bandlabels (Autodesk Fusion 360 design; units mm, degrees)
Autodesk Fusion 360 part; units mm, degrees
(part 1 of 2)
sketch "Sketch1" plane through (0, 0, 0) normal (0, 0, 1) x (1, 0, 0)
  line L0 (-15, -10) -> (-15, 8)
  line L1 (-15, 8) -> (15, 8)
  line L2 (15, 8) -> (15, -10)
  line L3 (15, -10) -> (-15, 8) construction
  line L4 (-15, -10) -> (15, 8) construction
  line L5 (15, -10) -> (15, -16.5)
  line L6 (6.1644, -16.5) -> (-15, -16.5)
  line L7 (-15, -10) -> (-15, -16.5)
  line L8 (6, 6) -> (-6, 6)
  line L9 (-6, 6) -> (-6, -6)
  line L10 (-6, -6) -> (6, -6)
  line L11 (6, -6) -> (6, 6)
  line L12 (6, 6) -> (-6, -6) construction
  line L13 (-6, 6) -> (6, -6) construction
  circle A0 centre (-11.792, 0) radius 1.75
  circle A1 centre (11.792, 0) radius 1.75
  line L14 (-15, -16.5) -> (15, -16.5)
  circle A2 centre (-11.792, -26) radius 1.75
  line L15 (-6, -32) -> (6, -32)
  line L16 (-6, -20) -> (-6, -32)
  line L17 (15, -36) -> (15, -42.5)
  line L18 (15, -18) -> (15, -36)
  line L19 (6, -32) -> (6, -20)
  line L20 (15, -36) -> (-15, -18) construction
  line L21 (-6, -20) -> (6, -32) construction
  line L22 (-15, -36) -> (15, -18) construction
  line L23 (-15, -36) -> (-15, -18)
  line L24 (6, -20) -> (-6, -20)
  line L25 (-15, -42.5) -> (15, -42.5)
  line L26 (6, -20) -> (-6, -32) construction
  circle A3 centre (11.792, -26) radius 1.75
  line L27 (-15, -36) -> (-15, -42.5)
  line L28 (6.1644, -42.5) -> (-15, -42.5)
  line L29 (-15, -18) -> (15, -18)
  line L30 (-48, -16.5) -> (-18, -16.5)
  line L31 (-18, -10) -> (-18, -16.5)
  circle A4 centre (-21.208, 0) radius 1.75
  line L32 (-27, -6) -> (-27, 6)
  line L33 (-27, 6) -> (-39, -6) construction
  line L34 (-48, -10) -> (-18, 8) construction
  line L35 (-39, 6) -> (-27, -6) construction
  circle A5 centre (-44.792, 0) radius 1.75
  line L36 (-18, -10) -> (-48, 8) construction
  line L37 (-48, -10) -> (-48, -16.5)
  line L38 (-39, 6) -> (-39, -6)
  line L39 (-27, 6) -> (-39, 6)
  line L40 (-26.8356, -16.5) -> (-48, -16.5)
  line L41 (-18, 8) -> (-18, -10)
  line L42 (-39, -6) -> (-27, -6)
  line L43 (-48, 8) -> (-18, 8)
  line L44 (-48, -10) -> (-48, 8)
  line L45 (-18, -36) -> (-48, -18) construction
  line L46 (-48, -36) -> (-48, -18)
  line L47 (-48, -42.5) -> (-18, -42.5)
  line L48 (-27, -32) -> (-27, -20)
  line L49 (-48, -36) -> (-48, -42.5)
  line L50 (-27, -20) -> (-39, -32) construction
  circle A6 centre (-44.792, -26) radius 1.75
  line L51 (-48, -18) -> (-18, -18)
  line L52 (-39, -20) -> (-39, -32)
  line L53 (-39, -20) -> (-27, -32) construction
  line L54 (-39, -32) -> (-27, -32)
  line L55 (-27, -20) -> (-39, -20)
  circle A7 centre (-21.208, -26) radius 1.75
  line L56 (-18, -18) -> (-18, -36)
  line L57 (-26.8356, -42.5) -> (-48, -42.5)
  line L58 (-18, -36) -> (-18, -42.5)
  line L59 (-48, -36) -> (-18, -18) construction
  line L60 (38, -6) -> (38, 6)
  line L61 (26, 6) -> (38, -6) construction
  line L62 (38, 6) -> (26, -6) construction
  circle A8 centre (20.208, 0) radius 1.75
  circle A9 centre (43.792, 0) radius 1.75
  line L63 (38, 6) -> (26, 6)
  line L64 (26, -6) -> (38, -6)
  line L65 (47, -10) -> (47, -16.5)
  line L66 (17, 8) -> (47, 8)
  line L67 (17, -10) -> (47, 8) construction
  line L68 (47, 8) -> (47, -10)
  line L69 (47, -10) -> (17, 8) construction
  line L70 (17, -16.5) -> (47, -16.5)
  line L71 (17, -10) -> (17, -16.5)
  line L72 (17, -10) -> (17, 8)
  line L73 (38.1644, -16.5) -> (17, -16.5)
  line L74 (26, 6) -> (26, -6)
  line L75 (17, -36) -> (47, -18) construction
  line L76 (47, -36) -> (17, -18) construction
  line L77 (47, -36) -> (47, -42.5)
  line L78 (38.1644, -42.5) -> (17, -42.5)
  line L79 (17, -36) -> (17, -42.5)
  circle A10 centre (43.792, -26) radius 1.75
  line L80 (17, -18) -> (47, -18)
  line L81 (38, -32) -> (38, -20)
  circle A11 centre (20.208, -26) radius 1.75
  line L82 (38, -20) -> (26, -32) construction
  line L83 (26, -32) -> (38, -32)
  line L84 (26, -20) -> (26, -32)
  line L85 (26, -20) -> (38, -32) construction
  line L86 (38, -20) -> (26, -20)
  line L87 (47, -18) -> (47, -36)
  line L88 (17, -36) -> (17, -18)
  line L89 (17, -42.5) -> (47, -42.5)
  line L90 (-18, -63) -> (-18, -69.5)
  line L91 (-27, -47) -> (-39, -59) construction
  line L92 (-48, -63) -> (-18, -45) construction
  circle A12 centre (-21.208, -53) radius 1.75
  line L93 (-48, -63) -> (-48, -45)
  line L94 (-48, -69.5) -> (-18, -69.5)
  line L95 (-18, -63) -> (-48, -45) construction
  line L96 (-39, -47) -> (-39, -59)
  line L97 (-26.8356, -69.5) -> (-48, -69.5)
  line L98 (-48, -45) -> (-18, -45)
  line L99 (-27, -47) -> (-39, -47)
  line L100 (-18, -45) -> (-18, -63)
  circle A13 centre (-44.792, -53) radius 1.75
  line L101 (-48, -63) -> (-48, -69.5)
  line L102 (-27, -59) -> (-27, -47)
  line L103 (-39, -47) -> (-27, -59) construction
  line L104 (-39, -59) -> (-27, -59)
  line L105 (-42.7356, -14.4017) -> (-42.7356, -14.9918)
  line L106 (-42.7356, -14.9918) -> (-46.0406, -14.9918)
  spline S0 degree 2 poles (-46.0406, -14.9918) (-46.0474, -14.7701) (-45.9689, -14.5655) knots 0 0 0 1 1 1
  spline S1 degree 2 poles (-45.9689, -14.5655) (-45.8427, -14.2278) (-45.5648, -13.9004) knots 0 0 0 1 1 1
  spline S2 degree 2 poles (-45.5648, -13.9004) (-45.2868, -13.573) (-44.7616, -13.1432) knots 0 0 0 1 1 1
  spline S3 degree 2 poles (-44.7616, -13.1432) (-43.9464, -12.4747) (-43.6599, -12.0842) knots 0 0 0 1 1 1
  spline S4 degree 2 poles (-43.6599, -12.0842) (-43.3734, -11.6937) (-43.3734, -11.3458) knots 0 0 0 1 1 1
  spline S5 degree 2 poles (-43.3734, -11.3458) (-43.3734, -10.9809) (-43.6344, -10.7302) knots 0 0 0 1 1 1
  spline S6 degree 2 poles (-43.6344, -10.7302) (-43.8953, -10.4795) (-44.3148, -10.4795) knots 0 0 0 1 1 1
  spline S7 degree 2 poles (-44.3148, -10.4795) (-44.7582, -10.4795) (-45.0242, -10.7455) knots 0 0 0 1 1 1
  spline S8 degree 2 poles (-45.0242, -10.7455) (-45.2902, -11.0116) (-45.2936, -11.4822) knots 0 0 0 1 1 1
  line L107 (-45.2936, -11.4822) -> (-45.9246, -11.4174)
  spline S9 degree 2 poles (-45.9246, -11.4174) (-45.8598, -10.7114) (-45.4369, -10.3414) knots 0 0 0 1 1 1
  spline S10 degree 2 poles (-45.4369, -10.3414) (-45.014, -9.9713) (-44.3011, -9.9713) knots 0 0 0 1 1 1
  spline S11 degree 2 poles (-44.3011, -9.9713) (-43.5815, -9.9713) (-43.162, -10.3704) knots 0 0 0 1 1 1
  spline S12 degree 2 poles (-43.162, -10.3704) (-42.7425, -10.7694) (-42.7425, -11.3594) knots 0 0 0 1 1 1
  spline S13 degree 2 poles (-42.7425, -11.3594) (-42.7425, -11.6596) (-42.8653, -11.9495) knots 0 0 0 1 1 1
  spline S14 degree 2 poles (-42.8653, -11.9495) (-42.988, -12.2394) (-43.2728, -12.56) knots 0 0 0 1 1 1
  spline S15 degree 2 poles (-43.2728, -12.56) (-43.5576, -12.8806) (-44.2193, -13.4399) knots 0 0 0 1 1 1
  spline S16 degree 2 poles (-44.2193, -13.4399) (-44.7718, -13.9038) (-44.9287, -14.0692) knots 0 0 0 1 1 1
  spline S17 degree 2 poles (-44.9287, -14.0692) (-45.0856, -14.2346) (-45.1879, -14.4017) knots 0 0 0 1 1 1
  line L108 (-45.1879, -14.4017) -> (-42.7356, -14.4017)
  spline S18 degree 2 poles (-42.0774, -12.5259) (-42.0774, -11.6391) (-41.8949, -11.0985) knots 0 0 0 1 1 1
  spline S19 degree 2 poles (-41.8949, -11.0985) (-41.7125, -10.5579) (-41.3526, -10.2646) knots 0 0 0 1 1 1
  spline S20 degree 2 poles (-41.3526, -10.2646) (-40.9928, -9.9713) (-40.4471, -9.9713) knots 0 0 0 1 1 1
  spline S21 degree 2 poles (-40.4471, -9.9713) (-40.0447, -9.9713) (-39.7411, -10.1333) knots 0 0 0 1 1 1
  spline S22 degree 2 poles (-39.7411, -10.1333) (-39.4376, -10.2953) (-39.2397, -10.6006) knots 0 0 0 1 1 1
  spline S23 degree 2 poles (-39.2397, -10.6006) (-39.0419, -10.9058) (-38.9294, -11.3441) knots 0 0 0 1 1 1
  spline S24 degree 2 poles (-38.9294, -11.3441) (-38.8168, -11.7824) (-38.8168, -12.5259) knots 0 0 0 1 1 1
  spline S25 degree 2 poles (-38.8168, -12.5259) (-38.8168, -13.4058) (-38.9976, -13.9464) knots 0 0 0 1 1 1
  spline S26 degree 2 poles (-38.9976, -13.9464) (-39.1784, -14.487) (-39.5382, -14.782) knots 0 0 0 1 1 1
  spline S27 degree 2 poles (-39.5382, -14.782) (-39.898, -15.077) (-40.4471, -15.077) knots 0 0 0 1 1 1
  spline S28 degree 2 poles (-40.4471, -15.077) (-41.1702, -15.077) (-41.5829, -14.5586) knots 0 0 0 1 1 1
  spline S29 degree 2 poles (-41.5829, -14.5586) (-42.0774, -13.9345) (-42.0774, -12.5259) knots 0 0 0 1 1 1
  spline S30 degree 2 poles (-41.4464, -12.5259) (-41.4464, -13.7571) (-41.1582, -14.1647) knots 0 0 0 1 1 1
  spline S31 degree 2 poles (-41.1582, -14.1647) (-40.87, -14.5723) (-40.4471, -14.5723) knots 0 0 0 1 1 1
  spline S32 degree 2 poles (-40.4471, -14.5723) (-40.0242, -14.5723) (-39.736, -14.163) knots 0 0 0 1 1 1
  spline S33 degree 2 poles (-39.736, -14.163) (-39.4478, -13.7537) (-39.4478, -12.5259) knots 0 0 0 1 1 1
  spline S34 degree 2 poles (-39.4478, -12.5259) (-39.4478, -11.2912) (-39.736, -10.8854) knots 0 0 0 1 1 1
  spline S35 degree 2 poles (-39.736, -10.8854) (-40.0242, -10.4795) (-40.4539, -10.4795) knots 0 0 0 1 1 1
  spline S36 degree 2 poles (-40.4539, -10.4795) (-40.8769, -10.4795) (-41.1292, -10.8376) knots 0 0 0 1 1 1
  spline S37 degree 2 poles (-41.1292, -10.8376) (-41.4464, -11.2946) (-41.4464, -12.5259) knots 0 0 0 1 1 1
  line L109 (-38.4826, -15.077) -> (-37.0331, -9.9065)
  line L110 (-37.0331, -9.9065) -> (-36.5419, -9.9065)
  line L111 (-36.5419, -9.9065) -> (-37.988, -15.077)
  line L112 (-37.988, -15.077) -> (-38.4826, -15.077)
  line L113 (-34.2841, -14.9918) -> (-34.2841, -13.7946)
  line L114 (-34.2841, -13.7946) -> (-36.4532, -13.7946)
  line L115 (-36.4532, -13.7946) -> (-36.4532, -13.2319)
  line L116 (-36.4532, -13.2319) -> (-34.1715, -9.9918)
  line L117 (-34.1715, -9.9918) -> (-33.6702, -9.9918)
  line L118 (-33.6702, -9.9918) -> (-33.6702, -13.2319)
  line L119 (-33.6702, -13.2319) -> (-32.9949, -13.2319)
  line L120 (-32.9949, -13.2319) -> (-32.9949, -13.7946)
  line L121 (-32.9949, -13.7946) -> (-33.6702, -13.7946)
  line L122 (-33.6702, -13.7946) -> (-33.6702, -14.9918)
  line L123 (-33.6702, -14.9918) -> (-34.2841, -14.9918)
  line L124 (-34.2841, -13.2319) -> (-34.2841, -10.9775)
  line L125 (-34.2841, -10.9775) -> (-35.8496, -13.2319)
  line L126 (-35.8496, -13.2319) -> (-34.2841, -13.2319)
  spline S38 degree 2 poles (-32.3673, -12.5259) (-32.3673, -11.6391) (-32.1848, -11.0985) knots 0 0 0 1 1 1
  spline S39 degree 2 poles (-32.1848, -11.0985) (-32.0024, -10.5579) (-31.6425, -10.2646) knots 0 0 0 1 1 1
  spline S40 degree 2 poles (-31.6425, -10.2646) (-31.2827, -9.9713) (-30.737, -9.9713) knots 0 0 0 1 1 1
  spline S41 degree 2 poles (-30.737, -9.9713) (-30.3346, -9.9713) (-30.031, -10.1333) knots 0 0 0 1 1 1
  spline S42 degree 2 poles (-30.031, -10.1333) (-29.7275, -10.2953) (-29.5296, -10.6006) knots 0 0 0 1 1 1
  spline S43 degree 2 poles (-29.5296, -10.6006) (-29.3318, -10.9058) (-29.2193, -11.3441) knots 0 0 0 1 1 1
  spline S44 degree 2 poles (-29.2193, -11.3441) (-29.1067, -11.7824) (-29.1067, -12.5259) knots 0 0 0 1 1 1
  spline S45 degree 2 poles (-29.1067, -12.5259) (-29.1067, -13.4058) (-29.2875, -13.9464) knots 0 0 0 1 1 1
  spline S46 degree 2 poles (-29.2875, -13.9464) (-29.4683, -14.487) (-29.8281, -14.782) knots 0 0 0 1 1 1
  spline S47 degree 2 poles (-29.8281, -14.782) (-30.1879, -15.077) (-30.737, -15.077) knots 0 0 0 1 1 1
  spline S48 degree 2 poles (-30.737, -15.077) (-31.4601, -15.077) (-31.8728, -14.5586) knots 0 0 0 1 1 1
  spline S49 degree 2 poles (-31.8728, -14.5586) (-32.3673, -13.9345) (-32.3673, -12.5259) knots 0 0 0 1 1 1
  spline S50 degree 2 poles (-31.7363, -12.5259) (-31.7363, -13.7571) (-31.4481, -14.1647) knots 0 0 0 1 1 1
  spline S51 degree 2 poles (-31.4481, -14.1647) (-31.1599, -14.5723) (-30.737, -14.5723) knots 0 0 0 1 1 1
  spline S52 degree 2 poles (-30.737, -14.5723) (-30.3141, -14.5723) (-30.0259, -14.163) knots 0 0 0 1 1 1
  spline S53 degree 2 poles (-30.0259, -14.163) (-29.7377, -13.7537) (-29.7377, -12.5259) knots 0 0 0 1 1 1
  spline S54 degree 2 poles (-29.7377, -12.5259) (-29.7377, -11.2912) (-30.0259, -10.8854) knots 0 0 0 1 1 1
  spline S55 degree 2 poles (-30.0259, -10.8854) (-30.3141, -10.4795) (-30.7438, -10.4795) knots 0 0 0 1 1 1
  spline S56 degree 2 poles (-30.7438, -10.4795) (-31.1668, -10.4795) (-31.4191, -10.8376) knots 0 0 0 1 1 1
  spline S57 degree 2 poles (-31.4191, -10.8376) (-31.7363, -11.2946) (-31.7363, -12.5259) knots 0 0 0 1 1 1
  line L127 (-28.7725, -15.077) -> (-27.323, -9.9065)
  line L128 (-27.323, -9.9065) -> (-26.8318, -9.9065)
  line L129 (-26.8318, -9.9065) -> (-28.2779, -15.077)
  line L130 (-28.2779, -15.077) -> (-28.7725, -15.077)
  line L131 (-23.3564, -11.2162) -> (-23.9669, -11.264)
  spline S58 degree 2 poles (-23.9669, -11.264) (-24.0487, -10.9024) (-24.1988, -10.7387) knots 0 0 0 1 1 1
  spline S59 degree 2 poles (-24.1988, -10.7387) (-24.4478, -10.4761) (-24.8127, -10.4761) knots 0 0 0 1 1 1
  spline S60 degree 2 poles (-24.8127, -10.4761) (-25.106, -10.4761) (-25.3277, -10.6398) knots 0 0 0 1 1 1
  spline S61 degree 2 poles (-25.3277, -10.6398) (-25.6176, -10.8513) (-25.7848, -11.2571) knots 0 0 0 1 1 1
  spline S62 degree 2 poles (-25.7848, -11.2571) (-25.9519, -11.663) (-25.9587, -12.4133) knots 0 0 0 1 1 1
  spline S63 degree 2 poles (-25.9587, -12.4133) (-25.737, -12.0757) (-25.4164, -11.912) knots 0 0 0 1 1 1
  spline S64 degree 2 poles (-25.4164, -11.912) (-25.0958, -11.7483) (-24.7445, -11.7483) knots 0 0 0 1 1 1
  spline S65 degree 2 poles (-24.7445, -11.7483) (-24.1306, -11.7483) (-23.6992, -12.2002) knots 0 0 0 1 1 1
  spline S66 degree 2 poles (-23.6992, -12.2002) (-23.2677, -12.6521) (-23.2677, -13.3683) knots 0 0 0 1 1 1
  spline S67 degree 2 poles (-23.2677, -13.3683) (-23.2677, -13.839) (-23.4706, -14.2431) knots 0 0 0 1 1 1
  spline S68 degree 2 poles (-23.4706, -14.2431) (-23.6736, -14.6473) (-24.0283, -14.8622) knots 0 0 0 1 1 1
  spline S69 degree 2 poles (-24.0283, -14.8622) (-24.383, -15.077) (-24.8332, -15.077) knots 0 0 0 1 1 1
  spline S70 degree 2 poles (-24.8332, -15.077) (-25.6006, -15.077) (-26.0849, -14.5126) knots 0 0 0 1 1 1
  spline S71 degree 2 poles (-26.0849, -14.5126) (-26.5692, -13.9481) (-26.5692, -12.6521) knots 0 0 0 1 1 1
  spline S72 degree 2 poles (-26.5692, -12.6521) (-26.5692, -11.2026) (-26.0337, -10.5443) knots 0 0 0 1 1 1
  spline S73 degree 2 poles (-26.0337, -10.5443) (-25.5665, -9.9713) (-24.7752, -9.9713) knots 0 0 0 1 1 1
  spline S74 degree 2 poles (-24.7752, -9.9713) (-24.1852, -9.9713) (-23.8083, -10.3022) knots 0 0 0 1 1 1
  spline S75 degree 2 poles (-23.8083, -10.3022) (-23.4314, -10.633) (-23.3564, -11.2162) knots 0 0 0 1 1 1
  spline S76 degree 2 poles (-25.8632, -13.3717) (-25.8632, -13.6889) (-25.7285, -13.9788) knots 0 0 0 1 1 1
  spline S77 degree 2 poles (-25.7285, -13.9788) (-25.5938, -14.2687) (-25.3516, -14.4205) knots 0 0 0 1 1 1
  spline S78 degree 2 poles (-25.3516, -14.4205) (-25.1095, -14.5723) (-24.8434, -14.5723) knots 0 0 0 1 1 1
  spline S79 degree 2 poles (-24.8434, -14.5723) (-24.4546, -14.5723) (-24.1749, -14.2585) knots 0 0 0 1 1 1
  spline S80 degree 2 poles (-24.1749, -14.2585) (-23.8953, -13.9447) (-23.8953, -13.4058) knots 0 0 0 1 1 1
  spline S81 degree 2 poles (-23.8953, -13.4058) (-23.8953, -12.8874) (-24.1715, -12.589) knots 0 0 0 1 1 1
  spline S82 degree 2 poles (-24.1715, -12.589) (-24.4478, -12.2906) (-24.8673, -12.2906) knots 0 0 0 1 1 1
  spline S83 degree 2 poles (-24.8673, -12.2906) (-25.2834, -12.2906) (-25.5733, -12.589) knots 0 0 0 1 1 1
  spline S84 degree 2 poles (-25.5733, -12.589) (-25.8632, -12.8874) (-25.8632, -13.3717) knots 0 0 0 1 1 1
  spline S85 degree 2 poles (-22.6572, -12.5259) (-22.6572, -11.6391) (-22.4747, -11.0985) knots 0 0 0 1 1 1
  spline S86 degree 2 poles (-22.4747, -11.0985) (-22.2923, -10.5579) (-21.9324, -10.2646) knots 0 0 0 1 1 1
  spline S87 degree 2 poles (-21.9324, -10.2646) (-21.5726, -9.9713) (-21.0269, -9.9713) knots 0 0 0 1 1 1
  spline S88 degree 2 poles (-21.0269, -9.9713) (-20.6245, -9.9713) (-20.3209, -10.1333) knots 0 0 0 1 1 1
  spline S89 degree 2 poles (-20.3209, -10.1333) (-20.0174, -10.2953) (-19.8196, -10.6006) knots 0 0 0 1 1 1
  spline S90 degree 2 poles (-19.8196, -10.6006) (-19.6217, -10.9058) (-19.5092, -11.3441) knots 0 0 0 1 1 1
  spline S91 degree 2 poles (-19.5092, -11.3441) (-19.3966, -11.7824) (-19.3966, -12.5259) knots 0 0 0 1 1 1
  spline S92 degree 2 poles (-19.3966, -12.5259) (-19.3966, -13.4058) (-19.5774, -13.9464) knots 0 0 0 1 1 1
  spline S93 degree 2 poles (-19.5774, -13.9464) (-19.7582, -14.487) (-20.118, -14.782) knots 0 0 0 1 1 1
  spline S94 degree 2 poles (-20.118, -14.782) (-20.4778, -15.077) (-21.0269, -15.077) knots 0 0 0 1 1 1
  spline S95 degree 2 poles (-21.0269, -15.077) (-21.75, -15.077) (-22.1627, -14.5586) knots 0 0 0 1 1 1
  spline S96 degree 2 poles (-22.1627, -14.5586) (-22.6572, -13.9345) (-22.6572, -12.5259) knots 0 0 0 1 1 1
  spline S97 degree 2 poles (-22.0262, -12.5259) (-22.0262, -13.7571) (-21.738, -14.1647) knots 0 0 0 1 1 1
  spline S98 degree 2 poles (-21.738, -14.1647) (-21.4498, -14.5723) (-21.0269, -14.5723) knots 0 0 0 1 1 1
  spline S99 degree 2 poles (-21.0269, -14.5723) (-20.604, -14.5723) (-20.3158, -14.163) knots 0 0 0 1 1 1
  spline S100 degree 2 poles (-20.3158, -14.163) (-20.0276, -13.7537) (-20.0276, -12.5259) knots 0 0 0 1 1 1
  spline S101 degree 2 poles (-20.0276, -12.5259) (-20.0276, -11.2912) (-20.3158, -10.8854) knots 0 0 0 1 1 1
  spline S102 degree 2 poles (-20.3158, -10.8854) (-20.604, -10.4795) (-21.0337, -10.4795) knots 0 0 0 1 1 1
  spline S103 degree 2 poles (-21.0337, -10.4795) (-21.4567, -10.4795) (-21.709, -10.8376) knots 0 0 0 1 1 1
  spline S104 degree 2 poles (-21.709, -10.8376) (-22.0262, -11.2946) (-22.0262, -12.5259) knots 0 0 0 1 1 1
  line L132 (-5.9416, -14.912) -> (-6.5555, -14.912)
  line L133 (-6.5555, -14.912) -> (-6.5555, -11)
  spline S105 degree 2 poles (-6.5555, -11) (-6.7772, -11.2115) (-7.137, -11.4229) knots 0 0 0 1 1 1
  spline S106 degree 2 poles (-7.137, -11.4229) (-7.4968, -11.6344) (-7.7833, -11.7401) knots 0 0 0 1 1 1
  line L134 (-7.7833, -11.7401) -> (-7.7833, -11.1467)
  spline S107 degree 2 poles (-7.7833, -11.1467) (-7.2683, -10.9045) (-6.8829, -10.56) knots 0 0 0 1 1 1
  spline S108 degree 2 poles (-6.8829, -10.56) (-6.4975, -10.2156) (-6.3372, -9.8916) knots 0 0 0 1 1 1
  line L135 (-6.3372, -9.8916) -> (-5.9416, -9.8916)
  line L136 (-5.9416, -9.8916) -> (-5.9416, -14.912)
  line L137 (-4.3693, -13.6023) -> (-3.7246, -13.5478)
  spline S109 degree 2 poles (-3.7246, -13.5478) (-3.653, -14.0184) (-3.3921, -14.2555) knots 0 0 0 1 1 1
  spline S110 degree 2 poles (-3.3921, -14.2555) (-3.1312, -14.4925) (-2.7628, -14.4925) knots 0 0 0 1 1 1
  spline S111 degree 2 poles (-2.7628, -14.4925) (-2.3195, -14.4925) (-2.0125, -14.1583) knots 0 0 0 1 1 1
  spline S112 degree 2 poles (-2.0125, -14.1583) (-1.7055, -13.824) (-1.7055, -13.2715) knots 0 0 0 1 1 1
  spline S113 degree 2 poles (-1.7055, -13.2715) (-1.7055, -12.7463) (-2.0006, -12.4427) knots 0 0 0 1 1 1
  spline S114 degree 2 poles (-2.0006, -12.4427) (-2.2956, -12.1392) (-2.7731, -12.1392) knots 0 0 0 1 1 1
  spline S115 degree 2 poles (-2.7731, -12.1392) (-3.0698, -12.1392) (-3.3085, -12.2739) knots 0 0 0 1 1 1
  spline S116 degree 2 poles (-3.3085, -12.2739) (-3.5473, -12.4086) (-3.6837, -12.6235) knots 0 0 0 1 1 1
  line L138 (-3.6837, -12.6235) -> (-4.2601, -12.5484)
  line L139 (-4.2601, -12.5484) -> (-3.7758, -9.9802)
  line L140 (-3.7758, -9.9802) -> (-1.2894, -9.9802)
  line L141 (-1.2894, -9.9802) -> (-1.2894, -10.5669)
  line L142 (-1.2894, -10.5669) -> (-3.2847, -10.5669)
  line L143 (-3.2847, -10.5669) -> (-3.5541, -11.9107)
  spline S117 degree 2 poles (-3.5541, -11.9107) (-3.1039, -11.5969) (-2.6094, -11.5969) knots 0 0 0 1 1 1
  spline S118 degree 2 poles (-2.6094, -11.5969) (-1.9545, -11.5969) (-1.5043, -12.0505) knots 0 0 0 1 1 1
  spline S119 degree 2 poles (-1.5043, -12.0505) (-1.0541, -12.5041) (-1.0541, -13.2169) knots 0 0 0 1 1 1
  spline S120 degree 2 poles (-1.0541, -13.2169) (-1.0541, -13.8957) (-1.4497, -14.3902) knots 0 0 0 1 1 1
  spline S121 degree 2 poles (-1.4497, -14.3902) (-1.9307, -14.9973) (-2.7628, -14.9973) knots 0 0 0 1 1 1
  spline S122 degree 2 poles (-2.7628, -14.9973) (-3.445, -14.9973) (-3.8764, -14.6153) knots 0 0 0 1 1 1
  spline S123 degree 2 poles (-3.8764, -14.6153) (-4.3079, -14.2333) (-4.3693, -13.6023) knots 0 0 0 1 1 1
  line L144 (1.6266, -14.912) -> (1.6266, -11.2899)
  line L145 (1.6266, -11.2899) -> (2.1758, -11.2899)
  line L146 (2.1758, -11.2899) -> (2.1758, -11.7981)
  spline S124 degree 2 poles (2.1758, -11.7981) (2.3463, -11.5321) (2.6294, -11.3701) knots 0 0 0 1 1 1
  spline S125 degree 2 poles (2.6294, -11.3701) (2.9125, -11.2081) (3.274, -11.2081) knots 0 0 0 1 1 1
  spline S126 degree 2 poles (3.274, -11.2081) (3.6764, -11.2081) (3.9339, -11.3752) knots 0 0 0 1 1 1
  spline S127 degree 2 poles (3.9339, -11.3752) (4.1915, -11.5423) (4.2972, -11.8424) knots 0 0 0 1 1 1
  spline S128 degree 2 poles (4.2972, -11.8424) (4.7269, -11.2081) (5.4159, -11.2081) knots 0 0 0 1 1 1
  spline S129 degree 2 poles (5.4159, -11.2081) (5.9548, -11.2081) (6.2447, -11.5065) knots 0 0 0 1 1 1
  spline S130 degree 2 poles (6.2447, -11.5065) (6.5346, -11.8049) (6.5346, -12.4257) knots 0 0 0 1 1 1
  line L147 (6.5346, -12.4257) -> (6.5346, -14.912)
  line L148 (6.5346, -14.912) -> (5.9241, -14.912)
  line L149 (5.9241, -14.912) -> (5.9241, -12.6303)
  spline S131 degree 2 poles (5.9241, -12.6303) (5.9241, -12.262) (5.8644, -12.1) knots 0 0 0 1 1 1
  spline S132 degree 2 poles (5.8644, -12.1) (5.8047, -11.9379) (5.6478, -11.839) knots 0 0 0 1 1 1
  spline S133 degree 2 poles (5.6478, -11.839) (5.4909, -11.7401) (5.2794, -11.7401) knots 0 0 0 1 1 1
  spline S134 degree 2 poles (5.2794, -11.7401) (4.8975, -11.7401) (4.6451, -11.9942) knots 0 0 0 1 1 1
  spline S135 degree 2 poles (4.6451, -11.9942) (4.3927, -12.2483) (4.3927, -12.8077) knots 0 0 0 1 1 1
  line L150 (4.3927, -12.8077) -> (4.3927, -14.912)
  line L151 (4.3927, -14.912) -> (3.7788, -14.912)
  line L152 (3.7788, -14.912) -> (3.7788, -12.5587)
  spline S136 degree 2 poles (3.7788, -12.5587) (3.7788, -12.1494) (3.6287, -11.9448) knots 0 0 0 1 1 1
  spline S137 degree 2 poles (3.6287, -11.9448) (3.4786, -11.7401) (3.1376, -11.7401) knots 0 0 0 1 1 1
  spline S138 degree 2 poles (3.1376, -11.7401) (2.8784, -11.7401) (2.6584, -11.8766) knots 0 0 0 1 1 1
  spline S139 degree 2 poles (2.6584, -11.8766) (2.4384, -12.013) (2.3395, -12.2756) knots 0 0 0 1 1 1
  spline S140 degree 2 poles (2.3395, -12.2756) (2.2406, -12.5382) (2.2406, -13.0328) knots 0 0 0 1 1 1
  line L153 (2.2406, -13.0328) -> (2.2406, -14.912)
  line L154 (2.2406, -14.912) -> (1.6266, -14.912)
  line L155 (26.0584, -14.912) -> (25.4445, -14.912)
  line L156 (25.4445, -14.912) -> (25.4445, -11)
  spline S141 degree 2 poles (25.4445, -11) (25.2228, -11.2115) (24.863, -11.4229) knots 0 0 0 1 1 1
  spline S142 degree 2 poles (24.863, -11.4229) (24.5032, -11.6344) (24.2167, -11.7401) knots 0 0 0 1 1 1
  line L157 (24.2167, -11.7401) -> (24.2167, -11.1467)
  spline S143 degree 2 poles (24.2167, -11.1467) (24.7317, -10.9045) (25.1171, -10.56) knots 0 0 0 1 1 1
  spline S144 degree 2 poles (25.1171, -10.56) (25.5025, -10.2156) (25.6628, -9.8916) knots 0 0 0 1 1 1
  line L158 (25.6628, -9.8916) -> (26.0584, -9.8916)
  line L159 (26.0584, -9.8916) -> (26.0584, -14.912)
  line L160 (30.8572, -14.322) -> (30.8572, -14.912)
  line L161 (30.8572, -14.912) -> (27.5523, -14.912)
  spline S145 degree 2 poles (27.5523, -14.912) (27.5455, -14.6903) (27.6239, -14.4857) knots 0 0 0 1 1 1
  spline S146 degree 2 poles (27.6239, -14.4857) (27.7501, -14.148) (28.0281, -13.8206) knots 0 0 0 1 1 1
  spline S147 degree 2 poles (28.0281, -13.8206) (28.306, -13.4932) (28.8313, -13.0635) knots 0 0 0 1 1 1
  spline S148 degree 2 poles (28.8313, -13.0635) (29.6464, -12.395) (29.9329, -12.0045) knots 0 0 0 1 1 1
  spline S149 degree 2 poles (29.9329, -12.0045) (30.2194, -11.6139) (30.2194, -11.266) knots 0 0 0 1 1 1
  spline S150 degree 2 poles (30.2194, -11.266) (30.2194, -10.9011) (29.9585, -10.6504) knots 0 0 0 1 1 1
  spline S151 degree 2 poles (29.9585, -10.6504) (29.6976, -10.3997) (29.2781, -10.3997) knots 0 0 0 1 1 1
  spline S152 degree 2 poles (29.2781, -10.3997) (28.8347, -10.3997) (28.5687, -10.6658) knots 0 0 0 1 1 1
  spline S153 degree 2 poles (28.5687, -10.6658) (28.3026, -10.9318) (28.2992, -11.4025) knots 0 0 0 1 1 1
  line L162 (28.2992, -11.4025) -> (27.6683, -11.3377)
  spline S154 degree 2 poles (27.6683, -11.3377) (27.7331, -10.6317) (28.156, -10.2616) knots 0 0 0 1 1 1
  spline S155 degree 2 poles (28.156, -10.2616) (28.5789, -9.8916) (29.2917, -9.8916) knots 0 0 0 1 1 1
  spline S156 degree 2 poles (29.2917, -9.8916) (30.0114, -9.8916) (30.4309, -10.2906) knots 0 0 0 1 1 1
  spline S157 degree 2 poles (30.4309, -10.2906) (30.8504, -10.6896) (30.8504, -11.2797) knots 0 0 0 1 1 1
  spline S158 degree 2 poles (30.8504, -11.2797) (30.8504, -11.5798) (30.7276, -11.8697) knots 0 0 0 1 1 1
  spline S159 degree 2 poles (30.7276, -11.8697) (30.6048, -12.1596) (30.32, -12.4802) knots 0 0 0 1 1 1
  spline S160 degree 2 poles (30.32, -12.4802) (30.0352, -12.8008) (29.3736, -13.3602) knots 0 0 0 1 1 1
  spline S161 degree 2 poles (29.3736, -13.3602) (28.8211, -13.824) (28.6642, -13.9894) knots 0 0 0 1 1 1
  spline S162 degree 2 poles (28.6642, -13.9894) (28.5073, -14.1549) (28.405, -14.322) knots 0 0 0 1 1 1
  line L163 (28.405, -14.322) -> (30.8572, -14.322)
  line L164 (33.6266, -14.912) -> (33.6266, -11.2899)
  line L165 (33.6266, -11.2899) -> (34.1758, -11.2899)
  line L166 (34.1758, -11.2899) -> (34.1758, -11.7981)
  spline S163 degree 2 poles (34.1758, -11.7981) (34.3463, -11.5321) (34.6294, -11.3701) knots 0 0 0 1 1 1
  spline S164 degree 2 poles (34.6294, -11.3701) (34.9125, -11.2081) (35.274, -11.2081) knots 0 0 0 1 1 1
  spline S165 degree 2 poles (35.274, -11.2081) (35.6764, -11.2081) (35.9339, -11.3752) knots 0 0 0 1 1 1
  spline S166 degree 2 poles (35.9339, -11.3752) (36.1915, -11.5423) (36.2972, -11.8424) knots 0 0 0 1 1 1
  spline S167 degree 2 poles (36.2972, -11.8424) (36.7269, -11.2081) (37.4159, -11.2081) knots 0 0 0 1 1 1
  spline S168 degree 2 poles (37.4159, -11.2081) (37.9548, -11.2081) (38.2447, -11.5065) knots 0 0 0 1 1 1
  spline S169 degree 2 poles (38.2447, -11.5065) (38.5346, -11.8049) (38.5346, -12.4257) knots 0 0 0 1 1 1
  line L167 (38.5346, -12.4257) -> (38.5346, -14.912)
  line L168 (38.5346, -14.912) -> (37.9241, -14.912)
  line L169 (37.9241, -14.912) -> (37.9241, -12.6303)
  spline S170 degree 2 poles (37.9241, -12.6303) (37.9241, -12.262) (37.8644, -12.1) knots 0 0 0 1 1 1
  spline S171 degree 2 poles (37.8644, -12.1) (37.8047, -11.9379) (37.6478, -11.839) knots 0 0 0 1 1 1
  spline S172 degree 2 poles (37.6478, -11.839) (37.4909, -11.7401) (37.2794, -11.7401) knots 0 0 0 1 1 1
  spline S173 degree 2 poles (37.2794, -11.7401) (36.8975, -11.7401) (36.6451, -11.9942) knots 0 0 0 1 1 1
  spline S174 degree 2 poles (36.6451, -11.9942) (36.3927, -12.2483) (36.3927, -12.8077) knots 0 0 0 1 1 1
  line L170 (36.3927, -12.8077) -> (36.3927, -14.912)
  line L171 (36.3927, -14.912) -> (35.7788, -14.912)
  line L172 (35.7788, -14.912) -> (35.7788, -12.5587)
  spline S175 degree 2 poles (35.7788, -12.5587) (35.7788, -12.1494) (35.6287, -11.9448) knots 0 0 0 1 1 1
  spline S176 degree 2 poles (35.6287, -11.9448) (35.4786, -11.7401) (35.1376, -11.7401) knots 0 0 0 1 1 1
  spline S177 degree 2 poles (35.1376, -11.7401) (34.8784, -11.7401) (34.6584, -11.8766) knots 0 0 0 1 1 1
  spline S178 degree 2 poles (34.6584, -11.8766) (34.4384, -12.013) (34.3395, -12.2756) knots 0 0 0 1 1 1
  spline S179 degree 2 poles (34.3395, -12.2756) (34.2406, -12.5382) (34.2406, -13.0328) knots 0 0 0 1 1 1
  line L173 (34.2406, -13.0328) -> (34.2406, -14.912)
  line L174 (34.2406, -14.912) -> (33.6266, -14.912)
  line L175 (-38.9416, -40.912) -> (-39.5555, -40.912)
  line L176 (-39.5555, -40.912) -> (-39.5555, -37)
  spline S180 degree 2 poles (-39.5555, -37) (-39.7772, -37.2115) (-40.137, -37.4229) knots 0 0 0 1 1 1
  spline S181 degree 2 poles (-40.137, -37.4229) (-40.4968, -37.6344) (-40.7833, -37.7401) knots 0 0 0 1 1 1
  line L177 (-40.7833, -37.7401) -> (-40.7833, -37.1467)
  spline S182 degree 2 poles (-40.7833, -37.1467) (-40.2683, -36.9045) (-39.8829, -36.56) knots 0 0 0 1 1 1
  spline S183 degree 2 poles (-39.8829, -36.56) (-39.4975, -36.2156) (-39.3372, -35.8916) knots 0 0 0 1 1 1
  line L178 (-39.3372, -35.8916) -> (-38.9416, -35.8916)
  line L179 (-38.9416, -35.8916) -> (-38.9416, -40.912)
  line L180 (-37.3283, -36.5669) -> (-37.3283, -35.9768)
  line L181 (-37.3283, -35.9768) -> (-34.0916, -35.9768)
  line L182 (-34.0916, -35.9768) -> (-34.0916, -36.4543)
  spline S184 degree 2 poles (-34.0916, -36.4543) (-34.5691, -36.9625) (-35.0381, -37.8049) knots 0 0 0 1 1 1
  spline S185 degree 2 poles (-35.0381, -37.8049) (-35.507, -38.6474) (-35.7628, -39.5375) knots 0 0 0 1 1 1
  spline S186 degree 2 poles (-35.7628, -39.5375) (-35.947, -40.1651) (-35.9982, -40.912) knots 0 0 0 1 1 1
  line L183 (-35.9982, -40.912) -> (-36.6291, -40.912)
  spline S187 degree 2 poles (-36.6291, -40.912) (-36.6189, -40.322) (-36.3972, -39.4864) knots 0 0 0 1 1 1
  spline S188 degree 2 poles (-36.3972, -39.4864) (-36.1755, -38.6508) (-35.7611, -37.8748) knots 0 0 0 1 1 1
  spline S189 degree 2 poles (-35.7611, -37.8748) (-35.3467, -37.0989) (-34.8795, -36.5669) knots 0 0 0 1 1 1
  line L184 (-34.8795, -36.5669) -> (-37.3283, -36.5669)
  line L185 (-31.3734, -40.912) -> (-31.3734, -37.2899)
  line L186 (-31.3734, -37.2899) -> (-30.8242, -37.2899)
  line L187 (-30.8242, -37.2899) -> (-30.8242, -37.7981)
  spline S190 degree 2 poles (-30.8242, -37.7981) (-30.6537, -37.5321) (-30.3706, -37.3701) knots 0 0 0 1 1 1
  spline S191 degree 2 poles (-30.3706, -37.3701) (-30.0875, -37.2081) (-29.726, -37.2081) knots 0 0 0 1 1 1
  spline S192 degree 2 poles (-29.726, -37.2081) (-29.3236, -37.2081) (-29.0661, -37.3752) knots 0 0 0 1 1 1
  spline S193 degree 2 poles (-29.0661, -37.3752) (-28.8085, -37.5423) (-28.7028, -37.8424) knots 0 0 0 1 1 1
  spline S194 degree 2 poles (-28.7028, -37.8424) (-28.2731, -37.2081) (-27.5841, -37.2081) knots 0 0 0 1 1 1
  spline S195 degree 2 poles (-27.5841, -37.2081) (-27.0452, -37.2081) (-26.7553, -37.5065) knots 0 0 0 1 1 1
  spline S196 degree 2 poles (-26.7553, -37.5065) (-26.4654, -37.8049) (-26.4654, -38.4257) knots 0 0 0 1 1 1
  line L188 (-26.4654, -38.4257) -> (-26.4654, -40.912)
  line L189 (-26.4654, -40.912) -> (-27.0759, -40.912)
  line L190 (-27.0759, -40.912) -> (-27.0759, -38.6303)
  spline S197 degree 2 poles (-27.0759, -38.6303) (-27.0759, -38.262) (-27.1356, -38.1) knots 0 0 0 1 1 1
  spline S198 degree 2 poles (-27.1356, -38.1) (-27.1953, -37.9379) (-27.3522, -37.839) knots 0 0 0 1 1 1
  spline S199 degree 2 poles (-27.3522, -37.839) (-27.5091, -37.7401) (-27.7206, -37.7401) knots 0 0 0 1 1 1
  spline S200 degree 2 poles (-27.7206, -37.7401) (-28.1025, -37.7401) (-28.3549, -37.9942) knots 0 0 0 1 1 1
  spline S201 degree 2 poles (-28.3549, -37.9942) (-28.6073, -38.2483) (-28.6073, -38.8077) knots 0 0 0 1 1 1
  line L191 (-28.6073, -38.8077) -> (-28.6073, -40.912)
  line L192 (-28.6073, -40.912) -> (-29.2212, -40.912)
  line L193 (-29.2212, -40.912) -> (-29.2212, -38.5587)
  spline S202 degree 2 poles (-29.2212, -38.5587) (-29.2212, -38.1494) (-29.3713, -37.9448) knots 0 0 0 1 1 1
  spline S203 degree 2 poles (-29.3713, -37.9448) (-29.5214, -37.7401) (-29.8624, -37.7401) knots 0 0 0 1 1 1
  spline S204 degree 2 poles (-29.8624, -37.7401) (-30.1216, -37.7401) (-30.3416, -37.8766) knots 0 0 0 1 1 1
  spline S205 degree 2 poles (-30.3416, -37.8766) (-30.5616, -38.013) (-30.6605, -38.2756) knots 0 0 0 1 1 1
  spline S206 degree 2 poles (-30.6605, -38.2756) (-30.7594, -38.5382) (-30.7594, -39.0328) knots 0 0 0 1 1 1
  line L194 (-30.7594, -39.0328) -> (-30.7594, -40.912)
  line L195 (-30.7594, -40.912) -> (-31.3734, -40.912)
  line L196 (-7.7833, -39.5921) -> (-7.1694, -39.5103)
  spline S207 degree 2 poles (-7.1694, -39.5103) (-7.0637, -40.0321) (-6.8096, -40.2623) knots 0 0 0 1 1 1
  spline S208 degree 2 poles (-6.8096, -40.2623) (-6.5555, -40.4925) (-6.1905, -40.4925) knots 0 0 0 1 1 1
  spline S209 degree 2 poles (-6.1905, -40.4925) (-5.7574, -40.4925) (-5.459, -40.1924) knots 0 0 0 1 1 1
  spline S210 degree 2 poles (-5.459, -40.1924) (-5.1605, -39.8922) (-5.1605, -39.4489) knots 0 0 0 1 1 1
  spline S211 degree 2 poles (-5.1605, -39.4489) (-5.1605, -39.0259) (-5.4368, -38.7514) knots 0 0 0 1 1 1
  spline S212 degree 2 poles (-5.4368, -38.7514) (-5.7131, -38.4768) (-6.1394, -38.4768) knots 0 0 0 1 1 1
  spline S213 degree 2 poles (-6.1394, -38.4768) (-6.3133, -38.4768) (-6.5725, -38.545) knots 0 0 0 1 1 1
  line L197 (-6.5725, -38.545) -> (-6.5043, -38.0062)
  spline S214 degree 2 poles (-6.5043, -38.0062) (-6.4429, -38.013) (-6.4054, -38.013) knots 0 0 0 1 1 1
  spline S215 degree 2 poles (-6.4054, -38.013) (-6.0132, -38.013) (-5.6994, -37.8083) knots 0 0 0 1 1 1
  spline S216 degree 2 poles (-5.6994, -37.8083) (-5.3856, -37.6037) (-5.3856, -37.1774) knots 0 0 0 1 1 1
  spline S217 degree 2 poles (-5.3856, -37.1774) (-5.3856, -36.8397) (-5.6141, -36.618) knots 0 0 0 1 1 1
  spline S218 degree 2 poles (-5.6141, -36.618) (-5.8427, -36.3963) (-6.2042, -36.3963) knots 0 0 0 1 1 1
  spline S219 degree 2 poles (-6.2042, -36.3963) (-6.5623, -36.3963) (-6.801, -36.6214) knots 0 0 0 1 1 1
  spline S220 degree 2 poles (-6.801, -36.6214) (-7.0398, -36.8465) (-7.108, -37.2967) knots 0 0 0 1 1 1
  line L198 (-7.108, -37.2967) -> (-7.7219, -37.1876)
  spline S221 degree 2 poles (-7.7219, -37.1876) (-7.6094, -36.5703) (-7.2103, -36.2309) knots 0 0 0 1 1 1
  spline S222 degree 2 poles (-7.2103, -36.2309) (-6.8113, -35.8916) (-6.2178, -35.8916) knots 0 0 0 1 1 1
  spline S223 degree 2 poles (-6.2178, -35.8916) (-5.8085, -35.8916) (-5.4641, -36.0672) knots 0 0 0 1 1 1
  spline S224 degree 2 poles (-5.4641, -36.0672) (-5.1196, -36.2429) (-4.9371, -36.5464) knots 0 0 0 1 1 1
  spline S225 degree 2 poles (-4.9371, -36.5464) (-4.7547, -36.85) (-4.7547, -37.191) knots 0 0 0 1 1 1
  spline S226 degree 2 poles (-4.7547, -37.191) (-4.7547, -37.515) (-4.9286, -37.7811) knots 0 0 0 1 1 1
  spline S227 degree 2 poles (-4.9286, -37.7811) (-5.1025, -38.0471) (-5.4436, -38.204) knots 0 0 0 1 1 1
  spline S228 degree 2 poles (-5.4436, -38.204) (-5.0002, -38.3063) (-4.7547, -38.6286) knots 0 0 0 1 1 1
  spline S229 degree 2 poles (-4.7547, -38.6286) (-4.5091, -38.9509) (-4.5091, -39.4352) knots 0 0 0 1 1 1
  spline S230 degree 2 poles (-4.5091, -39.4352) (-4.5091, -40.0901) (-4.9866, -40.5454) knots 0 0 0 1 1 1
  spline S231 degree 2 poles (-4.9866, -40.5454) (-5.4641, -41.0007) (-6.194, -41.0007) knots 0 0 0 1 1 1
  spline S232 degree 2 poles (-6.194, -41.0007) (-6.8522, -41.0007) (-7.2871, -40.6085) knots 0 0 0 1 1 1
  spline S233 degree 2 poles (-7.2871, -40.6085) (-7.7219, -40.2163) (-7.7833, -39.5921) knots 0 0 0 1 1 1
  spline S234 degree 2 poles (-3.902, -38.4461) (-3.902, -37.5594) (-3.7195, -37.0188) knots 0 0 0 1 1 1
  spline S235 degree 2 poles (-3.7195, -37.0188) (-3.5371, -36.4782) (-3.1772, -36.1849) knots 0 0 0 1 1 1
  spline S236 degree 2 poles (-3.1772, -36.1849) (-2.8174, -35.8916) (-2.2717, -35.8916) knots 0 0 0 1 1 1
  spline S237 degree 2 poles (-2.2717, -35.8916) (-1.8693, -35.8916) (-1.5657, -36.0536) knots 0 0 0 1 1 1
  spline S238 degree 2 poles (-1.5657, -36.0536) (-1.2622, -36.2156) (-1.0643, -36.5208) knots 0 0 0 1 1 1
  spline S239 degree 2 poles (-1.0643, -36.5208) (-0.8665, -36.8261) (-0.754, -37.2643) knots 0 0 0 1 1 1
  spline S240 degree 2 poles (-0.754, -37.2643) (-0.6414, -37.7026) (-0.6414, -38.4461) knots 0 0 0 1 1 1
  spline S241 degree 2 poles (-0.6414, -38.4461) (-0.6414, -39.3261) (-0.8222, -39.8667) knots 0 0 0 1 1 1
  spline S242 degree 2 poles (-0.8222, -39.8667) (-1.003, -40.4072) (-1.3628, -40.7023) knots 0 0 0 1 1 1
  spline S243 degree 2 poles (-1.3628, -40.7023) (-1.7226, -40.9973) (-2.2717, -40.9973) knots 0 0 0 1 1 1
  spline S244 degree 2 poles (-2.2717, -40.9973) (-2.9948, -40.9973) (-3.4075, -40.4789) knots 0 0 0 1 1 1
  spline S245 degree 2 poles (-3.4075, -40.4789) (-3.902, -39.8547) (-3.902, -38.4461) knots 0 0 0 1 1 1
  spline S246 degree 2 poles (-3.271, -38.4461) (-3.271, -39.6774) (-2.9828, -40.0849) knots 0 0 0 1 1 1
  spline S247 degree 2 poles (-2.9828, -40.0849) (-2.6946, -40.4925) (-2.2717, -40.4925) knots 0 0 0 1 1 1
  spline S248 degree 2 poles (-2.2717, -40.4925) (-1.8488, -40.4925) (-1.5606, -40.0832) knots 0 0 0 1 1 1
  spline S249 degree 2 poles (-1.5606, -40.0832) (-1.2724, -39.674) (-1.2724, -38.4461) knots 0 0 0 1 1 1
  spline S250 degree 2 poles (-1.2724, -38.4461) (-1.2724, -37.2115) (-1.5606, -36.8056) knots 0 0 0 1 1 1
  spline S251 degree 2 poles (-1.5606, -36.8056) (-1.8488, -36.3997) (-2.2785, -36.3997) knots 0 0 0 1 1 1
  spline S252 degree 2 poles (-2.2785, -36.3997) (-2.7015, -36.3997) (-2.9538, -36.7579) knots 0 0 0 1 1 1
  spline S253 degree 2 poles (-2.9538, -36.7579) (-3.271, -37.2149) (-3.271, -38.4461) knots 0 0 0 1 1 1
  line L199 (2.0939, -40.912) -> (2.0939, -37.2899)
  line L200 (2.0939, -37.2899) -> (2.643, -37.2899)
  line L201 (2.643, -37.2899) -> (2.643, -37.7981)
  spline S254 degree 2 poles (2.643, -37.7981) (2.8136, -37.5321) (3.0966, -37.3701) knots 0 0 0 1 1 1
  spline S255 degree 2 poles (3.0966, -37.3701) (3.3797, -37.2081) (3.7412, -37.2081) knots 0 0 0 1 1 1
  spline S256 degree 2 poles (3.7412, -37.2081) (4.1437, -37.2081) (4.4012, -37.3752) knots 0 0 0 1 1 1
  spline S257 degree 2 poles (4.4012, -37.3752) (4.6587, -37.5423) (4.7644, -37.8424) knots 0 0 0 1 1 1
  spline S258 degree 2 poles (4.7644, -37.8424) (5.1942, -37.2081) (5.8831, -37.2081) knots 0 0 0 1 1 1
  spline S259 degree 2 poles (5.8831, -37.2081) (6.422, -37.2081) (6.7119, -37.5065) knots 0 0 0 1 1 1
  spline S260 degree 2 poles (6.7119, -37.5065) (7.0018, -37.8049) (7.0018, -38.4257) knots 0 0 0 1 1 1
  line L202 (7.0018, -38.4257) -> (7.0018, -40.912)
  line L203 (7.0018, -40.912) -> (6.3913, -40.912)
  line L204 (6.3913, -40.912) -> (6.3913, -38.6303)
  spline S261 degree 2 poles (6.3913, -38.6303) (6.3913, -38.262) (6.3316, -38.1) knots 0 0 0 1 1 1
  spline S262 degree 2 poles (6.3316, -38.1) (6.2719, -37.9379) (6.1151, -37.839) knots 0 0 0 1 1 1
  spline S263 degree 2 poles (6.1151, -37.839) (5.9582, -37.7401) (5.7467, -37.7401) knots 0 0 0 1 1 1
  spline S264 degree 2 poles (5.7467, -37.7401) (5.3647, -37.7401) (5.1123, -37.9942) knots 0 0 0 1 1 1
  spline S265 degree 2 poles (5.1123, -37.9942) (4.8599, -38.2483) (4.8599, -38.8077) knots 0 0 0 1 1 1
  line L205 (4.8599, -38.8077) -> (4.8599, -40.912)
  line L206 (4.8599, -40.912) -> (4.246, -40.912)
  line L207 (4.246, -40.912) -> (4.246, -38.5587)
  spline S266 degree 2 poles (4.246, -38.5587) (4.246, -38.1494) (4.096, -37.9448) knots 0 0 0 1 1 1
  spline S267 degree 2 poles (4.096, -37.9448) (3.9459, -37.7401) (3.6048, -37.7401) knots 0 0 0 1 1 1
  spline S268 degree 2 poles (3.6048, -37.7401) (3.3456, -37.7401) (3.1256, -37.8766) knots 0 0 0 1 1 1
  spline S269 degree 2 poles (3.1256, -37.8766) (2.9056, -38.013) (2.8067, -38.2756) knots 0 0 0 1 1 1
  spline S270 degree 2 poles (2.8067, -38.2756) (2.7078, -38.5382) (2.7078, -39.0328) knots 0 0 0 1 1 1
  line L208 (2.7078, -39.0328) -> (2.7078, -40.912)
  line L209 (2.7078, -40.912) -> (2.0939, -40.912)
  line L210 (26.0584, -40.912) -> (25.4445, -40.912)
  line L211 (25.4445, -40.912) -> (25.4445, -37)
  spline S271 degree 2 poles (25.4445, -37) (25.2228, -37.2115) (24.863, -37.4229) knots 0 0 0 1 1 1
  spline S272 degree 2 poles (24.863, -37.4229) (24.5032, -37.6344) (24.2167, -37.7401) knots 0 0 0 1 1 1
  line L212 (24.2167, -37.7401) -> (24.2167, -37.1467)
  spline S273 degree 2 poles (24.2167, -37.1467) (24.7317, -36.9045) (25.1171, -36.56) knots 0 0 0 1 1 1
  spline S274 degree 2 poles (25.1171, -36.56) (25.5025, -36.2156) (25.6628, -35.8916) knots 0 0 0 1 1 1
  line L213 (25.6628, -35.8916) -> (26.0584, -35.8916)
  line L214 (26.0584, -35.8916) -> (26.0584, -40.912)
  spline S275 degree 2 poles (27.6307, -38.4461) (27.6307, -37.5594) (27.8132, -37.0188) knots 0 0 0 1 1 1
  spline S276 degree 2 poles (27.8132, -37.0188) (27.9957, -36.4782) (28.3555, -36.1849) knots 0 0 0 1 1 1
  spline S277 degree 2 poles (28.3555, -36.1849) (28.7153, -35.8916) (29.261, -35.8916) knots 0 0 0 1 1 1
  spline S278 degree 2 poles (29.261, -35.8916) (29.6635, -35.8916) (29.967, -36.0536) knots 0 0 0 1 1 1
  spline S279 degree 2 poles (29.967, -36.0536) (30.2706, -36.2156) (30.4684, -36.5208) knots 0 0 0 1 1 1
  spline S280 degree 2 poles (30.4684, -36.5208) (30.6662, -36.8261) (30.7788, -37.2643) knots 0 0 0 1 1 1
  spline S281 degree 2 poles (30.7788, -37.2643) (30.8913, -37.7026) (30.8913, -38.4461) knots 0 0 0 1 1 1
  spline S282 degree 2 poles (30.8913, -38.4461) (30.8913, -39.3261) (30.7106, -39.8667) knots 0 0 0 1 1 1
  spline S283 degree 2 poles (30.7106, -39.8667) (30.5298, -40.4072) (30.17, -40.7023) knots 0 0 0 1 1 1
  spline S284 degree 2 poles (30.17, -40.7023) (29.8101, -40.9973) (29.261, -40.9973) knots 0 0 0 1 1 1
  spline S285 degree 2 poles (29.261, -40.9973) (28.538, -40.9973) (28.1253, -40.4789) knots 0 0 0 1 1 1
  spline S286 degree 2 poles (28.1253, -40.4789) (27.6307, -39.8547) (27.6307, -38.4461) knots 0 0 0 1 1 1
  spline S287 degree 2 poles (28.2617, -38.4461) (28.2617, -39.6774) (28.5499, -40.0849) knots 0 0 0 1 1 1
  spline S288 degree 2 poles (28.5499, -40.0849) (28.8381, -40.4925) (29.261, -40.4925) knots 0 0 0 1 1 1
  spline S289 degree 2 poles (29.261, -40.4925) (29.6839, -40.4925) (29.9721, -40.0832) knots 0 0 0 1 1 1
  spline S290 degree 2 poles (29.9721, -40.0832) (30.2603, -39.674) (30.2603, -38.4461) knots 0 0 0 1 1 1
  spline S291 degree 2 poles (30.2603, -38.4461) (30.2603, -37.2115) (29.9721, -36.8056) knots 0 0 0 1 1 1
  spline S292 degree 2 poles (29.9721, -36.8056) (29.6839, -36.3997) (29.2542, -36.3997) knots 0 0 0 1 1 1
  spline S293 degree 2 poles (29.2542, -36.3997) (28.8313, -36.3997) (28.5789, -36.7579) knots 0 0 0 1 1 1
  spline S294 degree 2 poles (28.5789, -36.7579) (28.2617, -37.2149) (28.2617, -38.4461) knots 0 0 0 1 1 1
  line L215 (33.6266, -40.912) -> (33.6266, -37.2899)
  line L216 (33.6266, -37.2899) -> (34.1758, -37.2899)
  line L217 (34.1758, -37.2899) -> (34.1758, -37.7981)
  spline S295 degree 2 poles (34.1758, -37.7981) (34.3463, -37.5321) (34.6294, -37.3701) knots 0 0 0 1 1 1
  spline S296 degree 2 poles (34.6294, -37.3701) (34.9125, -37.2081) (35.274, -37.2081) knots 0 0 0 1 1 1
  spline S297 degree 2 poles (35.274, -37.2081) (35.6764, -37.2081) (35.9339, -37.3752) knots 0 0 0 1 1 1
  spline S298 degree 2 poles (35.9339, -37.3752) (36.1915, -37.5423) (36.2972, -37.8424) knots 0 0 0 1 1 1
  spline S299 degree 2 poles (36.2972, -37.8424) (36.7269, -37.2081) (37.4159, -37.2081) knots 0 0 0 1 1 1
  spline S300 degree 2 poles (37.4159, -37.2081) (37.9548, -37.2081) (38.2447, -37.5065) knots 0 0 0 1 1 1
  spline S301 degree 2 poles (38.2447, -37.5065) (38.5346, -37.8049) (38.5346, -38.4257) knots 0 0 0 1 1 1
  line L218 (38.5346, -38.4257) -> (38.5346, -40.912)
  line L219 (38.5346, -40.912) -> (37.9241, -40.912)
  line L220 (37.9241, -40.912) -> (37.9241, -38.6303)
  spline S302 degree 2 poles (37.9241, -38.6303) (37.9241, -38.262) (37.8644, -38.1) knots 0 0 0 1 1 1
  spline S303 degree 2 poles (37.8644, -38.1) (37.8047, -37.9379) (37.6478, -37.839) knots 0 0 0 1 1 1
  spline S304 degree 2 poles (37.6478, -37.839) (37.4909, -37.7401) (37.2794, -37.7401) knots 0 0 0 1 1 1
  spline S305 degree 2 poles (37.2794, -37.7401) (36.8975, -37.7401) (36.6451, -37.9942) knots 0 0 0 1 1 1
  spline S306 degree 2 poles (36.6451, -37.9942) (36.3927, -38.2483) (36.3927, -38.8077) knots 0 0 0 1 1 1
  line L221 (36.3927, -38.8077) -> (36.3927, -40.912)
  line L222 (36.3927, -40.912) -> (35.7788, -40.912)
  line L223 (35.7788, -40.912) -> (35.7788, -38.5587)
  spline S307 degree 2 poles (35.7788, -38.5587) (35.7788, -38.1494) (35.6287, -37.9448) knots 0 0 0 1 1 1
  spline S308 degree 2 poles (35.6287, -37.9448) (35.4786, -37.7401) (35.1376, -37.7401) knots 0 0 0 1 1 1
  spline S309 degree 2 poles (35.1376, -37.7401) (34.8784, -37.7401) (34.6584, -37.8766) knots 0 0 0 1 1 1
  spline S310 degree 2 poles (34.6584, -37.8766) (34.4384, -38.013) (34.3395, -38.2756) knots 0 0 0 1 1 1
  spline S311 degree 2 poles (34.3395, -38.2756) (34.2406, -38.5382) (34.2406, -39.0328) knots 0 0 0 1 1 1
  line L224 (34.2406, -39.0328) -> (34.2406, -40.912)
  line L225 (34.2406, -40.912) -> (33.6266, -40.912)
  line L226 (-37.5705, -64.1364) -> (-38.181, -64.1842)
  spline S312 degree 2 poles (-38.181, -64.1842) (-38.2628, -63.8227) (-38.4129, -63.659) knots 0 0 0 1 1 1
  spline S313 degree 2 poles (-38.4129, -63.659) (-38.6619, -63.3963) (-39.0268, -63.3963) knots 0 0 0 1 1 1
  spline S314 degree 2 poles (-39.0268, -63.3963) (-39.3201, -63.3963) (-39.5418, -63.56) knots 0 0 0 1 1 1
  spline S315 degree 2 poles (-39.5418, -63.56) (-39.8317, -63.7715) (-39.9989, -64.1774) knots 0 0 0 1 1 1
  spline S316 degree 2 poles (-39.9989, -64.1774) (-40.166, -64.5832) (-40.1728, -65.3336) knots 0 0 0 1 1 1
  spline S317 degree 2 poles (-40.1728, -65.3336) (-39.9511, -64.9959) (-39.6305, -64.8322) knots 0 0 0 1 1 1
  spline S318 degree 2 poles (-39.6305, -64.8322) (-39.3099, -64.6685) (-38.9586, -64.6685) knots 0 0 0 1 1 1
  spline S319 degree 2 poles (-38.9586, -64.6685) (-38.3447, -64.6685) (-37.9133, -65.1204) knots 0 0 0 1 1 1
  spline S320 degree 2 poles (-37.9133, -65.1204) (-37.4818, -65.5723) (-37.4818, -66.2886) knots 0 0 0 1 1 1
  spline S321 degree 2 poles (-37.4818, -66.2886) (-37.4818, -66.7592) (-37.6847, -67.1634) knots 0 0 0 1 1 1
  spline S322 degree 2 poles (-37.6847, -67.1634) (-37.8877, -67.5675) (-38.2424, -67.7824) knots 0 0 0 1 1 1
  spline S323 degree 2 poles (-38.2424, -67.7824) (-38.5971, -67.9973) (-39.0473, -67.9973) knots 0 0 0 1 1 1
  spline S324 degree 2 poles (-39.0473, -67.9973) (-39.8147, -67.9973) (-40.299, -67.4328) knots 0 0 0 1 1 1
  spline S325 degree 2 poles (-40.299, -67.4328) (-40.7833, -66.8684) (-40.7833, -65.5723) knots 0 0 0 1 1 1
  spline S326 degree 2 poles (-40.7833, -65.5723) (-40.7833, -64.1228) (-40.2478, -63.4645) knots 0 0 0 1 1 1
  spline S327 degree 2 poles (-40.2478, -63.4645) (-39.7806, -62.8916) (-38.9893, -62.8916) knots 0 0 0 1 1 1
  spline S328 degree 2 poles (-38.9893, -62.8916) (-38.3993, -62.8916) (-38.0224, -63.2224) knots 0 0 0 1 1 1
  spline S329 degree 2 poles (-38.0224, -63.2224) (-37.6455, -63.5532) (-37.5705, -64.1364) knots 0 0 0 1 1 1
  spline S330 degree 2 poles (-40.0773, -66.292) (-40.0773, -66.6092) (-39.9426, -66.8991) knots 0 0 0 1 1 1
  spline S331 degree 2 poles (-39.9426, -66.8991) (-39.8079, -67.189) (-39.5657, -67.3407) knots 0 0 0 1 1 1
  spline S332 degree 2 poles (-39.5657, -67.3407) (-39.3236, -67.4925) (-39.0575, -67.4925) knots 0 0 0 1 1 1
  spline S333 degree 2 poles (-39.0575, -67.4925) (-38.6687, -67.4925) (-38.389, -67.1787) knots 0 0 0 1 1 1
  spline S334 degree 2 poles (-38.389, -67.1787) (-38.1094, -66.865) (-38.1094, -66.3261) knots 0 0 0 1 1 1
  spline S335 degree 2 poles (-38.1094, -66.3261) (-38.1094, -65.8077) (-38.3856, -65.5092) knots 0 0 0 1 1 1
  spline S336 degree 2 poles (-38.3856, -65.5092) (-38.6619, -65.2108) (-39.0814, -65.2108) knots 0 0 0 1 1 1
  spline S337 degree 2 poles (-39.0814, -65.2108) (-39.4975, -65.2108) (-39.7874, -65.5092) knots 0 0 0 1 1 1
  spline S338 degree 2 poles (-39.7874, -65.5092) (-40.0773, -65.8077) (-40.0773, -66.292) knots 0 0 0 1 1 1
  line L227 (-34.7601, -67.912) -> (-34.7601, -64.2899)
  line L228 (-34.7601, -64.2899) -> (-34.211, -64.2899)
  line L229 (-34.211, -64.2899) -> (-34.211, -64.7981)
  spline S339 degree 2 poles (-34.211, -64.7981) (-34.0405, -64.5321) (-33.7574, -64.3701) knots 0 0 0 1 1 1
  spline S340 degree 2 poles (-33.7574, -64.3701) (-33.4743, -64.2081) (-33.1128, -64.2081) knots 0 0 0 1 1 1
  spline S341 degree 2 poles (-33.1128, -64.2081) (-32.7103, -64.2081) (-32.4528, -64.3752) knots 0 0 0 1 1 1
  spline S342 degree 2 poles (-32.4528, -64.3752) (-32.1953, -64.5423) (-32.0896, -64.8424) knots 0 0 0 1 1 1
  spline S343 degree 2 poles (-32.0896, -64.8424) (-31.6598, -64.2081) (-30.9709, -64.2081) knots 0 0 0 1 1 1
  spline S344 degree 2 poles (-30.9709, -64.2081) (-30.432, -64.2081) (-30.1421, -64.5065) knots 0 0 0 1 1 1
  spline S345 degree 2 poles (-30.1421, -64.5065) (-29.8522, -64.8049) (-29.8522, -65.4257) knots 0 0 0 1 1 1
  line L230 (-29.8522, -65.4257) -> (-29.8522, -67.912)
  line L231 (-29.8522, -67.912) -> (-30.4627, -67.912)
  line L232 (-30.4627, -67.912) -> (-30.4627, -65.6303)
  spline S346 degree 2 poles (-30.4627, -65.6303) (-30.4627, -65.262) (-30.5224, -65.1) knots 0 0 0 1 1 1
  spline S347 degree 2 poles (-30.5224, -65.1) (-30.5821, -64.9379) (-30.739, -64.839) knots 0 0 0 1 1 1
  spline S348 degree 2 poles (-30.739, -64.839) (-30.8959, -64.7401) (-31.1073, -64.7401) knots 0 0 0 1 1 1
  spline S349 degree 2 poles (-31.1073, -64.7401) (-31.4893, -64.7401) (-31.7417, -64.9942) knots 0 0 0 1 1 1
  spline S350 degree 2 poles (-31.7417, -64.9942) (-31.9941, -65.2483) (-31.9941, -65.8077) knots 0 0 0 1 1 1
  line L233 (-31.9941, -65.8077) -> (-31.9941, -67.912)
  line L234 (-31.9941, -67.912) -> (-32.608, -67.912)
  line L235 (-32.608, -67.912) -> (-32.608, -65.5587)
  spline S351 degree 2 poles (-32.608, -65.5587) (-32.608, -65.1494) (-32.7581, -64.9448) knots 0 0 0 1 1 1
  spline S352 degree 2 poles (-32.7581, -64.9448) (-32.9081, -64.7401) (-33.2492, -64.7401) knots 0 0 0 1 1 1
  spline S353 degree 2 poles (-33.2492, -64.7401) (-33.5084, -64.7401) (-33.7284, -64.8766) knots 0 0 0 1 1 1